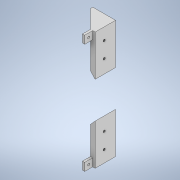
# Autodesk Inventor part: usb_battery_pocket_2
Saved by Autodesk Inventor 2021.3 (Build 253353010, 353A)
## iProperties
Created: 2021-10-31
Part Number: usb_battery_pocket_2
Material: Generic
Document SubType Name: Modeling
Designer: jesse
Density: 1 g/cm^3
Appearance: Default
Author: jesse
Autodesk Inventor part; units mm, degrees
ref_plane "YZ Plane" through (0, 0, 0) normal (1, 0, 0) x (0, 1, 0)
ref_plane "XZ Plane" through (0, 0, 0) normal (0, 1, 0) x (-1, 0, 0)
ref_plane "XY Plane" through (0, 0, 0) normal (0, 0, 1) x (1, 0, 0)
sketch "Sketch1" plane through (0, 0, 0) normal (0, 1, 0) x (-1, 0, 0)
  line L0 (0.4379, 4.9107) -> (0.4379, -5.0893)
  line L1 (0.4379, -5.0893) -> (-2.7621, -5.0893)
  line L2 (-2.7621, -5.0893) -> (-2.7621, -31.0893)
  line L3 (-2.7621, -31.0893) -> (26.2379, -31.0893)
  line L4 (26.2379, -31.0893) -> (26.2379, -28.0893)
  line L5 (26.2379, -28.0893) -> (0.2379, -28.0893)
  line L6 (0.2379, -28.0893) -> (0.2379, -8.0893)
  line L7 (0.2379, -8.0893) -> (3.2379, -8.0893)
  line L8 (3.2379, -8.0893) -> (3.2379, 4.9107)
  line L9 (3.2379, 4.9107) -> (0.4379, 4.9107)
  circle A0 centre (11.7379, -16.5893) radius 11.5
  line L10 (3.2379, -8.0893) -> (3.2379, -8.8433)
  line L11 (3.2379, -5.0893) -> (26.2379, -28.0893)
  point P0 (0, 0)
  point P1 (11.7379, -28.0893)
  point P2 (5.2457, -7.0971)
  dimension "d61" = 23
  dimension "d0" = 20
  dimension "d1" = 3
  dimension "d2" = 3
  dimension "d3" = 2.8
  dimension "d4" = 10
  dimension "d5" = 3
  dimension "d7" = 3.2
  dimension "d8" = 23
  constraints: 24 end point, 9 perpendicular, 3 vertical, 1 horizontal, 1 point on line, 3 other
  measures "d0" distance of L5.end L6.end
  measures "d1" distance between parallel lines of L2 L6
  measures "d2" distance between parallel lines of L7 L1
  measures "d3" distance between parallel lines of L0 L8
  measures "d4" distance of L0.start L0.end
  measures "d5" distance between parallel lines of L3 L5
  measures "d7" distance of L0.end L1.end
  measures "d8" horizontal distance of L11.start L4.end
extrude "Extrusion1" add sketch "Sketch1" along normal blind 150 contours L9 L8 L7 L6 L5 L4 L3 L2 L1 L0 | L11 A0 L10 L8 | L10 A0 L6 L7 | A0 L5 L6
sketch "Sketch2" plane through (2.7621, 0, -31.0893) normal (0, 0, -1) x (-1, 0, 0)
  line L0 (29, 0) -> (29, 150) projected
  line L1 (29, 130) -> (0, 98)
  line L2 (0, 0) -> (0, 150) projected
  line L3 (29, 20) -> (0, 52)
  line L4 (0, 0) -> (29, 0) projected
  point P0 (2.7621, 0)
  dimension "d11" = 20
  dimension "d12" = 20
  dimension "d13" = 32
  dimension "d14" = 32
  constraints: 4 end point, 4 point on line
  measures "d11" distance from line of L4 L3.start
  measures "d12" distance of L1.start L0.end
  measures "d13" vertical distance of L1.start L1.end
  measures "d14" vertical distance of L3.start L3.end
extrude "Extrusion2" cut sketch "Sketch2" against normal blind 150 contours L3 L2 L1 L0
sketch "Sketch3" plane through (-3.2379, 150, -5.0893) normal (-1, 0, 0) x (0, 0, 1)
  line L0 (0, 0) -> (10, 0) projected
  line L1 (0, -150) -> (0, -104.6207) projected
  line L2 (10, 0) -> (0, 0)
  line L3 (0, 0) -> (0, -150)
  line L4 (0, -150) -> (10, -150)
  line L5 (10, -150) -> (10, 0)
  line L6 (10, -48.469) -> (10, 0) projected
  line L7 (10, -10) -> (0, -10)
  line L8 (10, -150) -> (10, -104.6207) projected
  line L9 (10, -140) -> (0, -140)
  circle A0 centre (5, -5) radius 1.4
  circle A1 centre (5, -145) radius 1.4
  point P0 (5.0893, -150)
  point P1 (0, -140)
  dimension "d17" = 10
  dimension "d18" = 10
  dimension "d19" = 2.8
  dimension "d20" = 2.8
  dimension "d21" = 5
  dimension "d22" = 5
  dimension "d23" = 5
  dimension "d24" = 5
  constraints: 12 end point, 4 point on line, 3 perpendicular, 2 centre point, 2 parallel, 1 horizontal
  measures "d17" distance between parallel lines of L7 L0
  measures "d18" distance between parallel lines of L4 L9
  measures "d19" diameter of A0
  measures "d20" diameter of A1
  measures "d21" distance from line of L3 A0.centre
  measures "d22" distance from line of L0 A0.centre
  measures "d23" distance from line of L4 A1.centre
  measures "d24" distance from line of L1 A1.centre
extrude "Extrusion3" cut sketch "Sketch3" against normal blind 150 contours L7 L5 L9 L1 L3 | A0 | A1
sketch "Sketch5" plane through (2.7621, 150, -5.0893) normal (1, 0, 0) x (0, 0, -1)
  line L0 (2.0078, 0) -> (0, 0) projected
  line L1 (23, -36) -> (23, 0) projected
  line L2 (2.0078, 0) -> (23, 0)
  line L3 (23, 0) -> (23, -3)
  line L4 (23, -3) -> (2.0078, -3)
  line L5 (2.0078, -3) -> (2.0078, 0)
  line L6 (2.0078, -150) -> (2.0078, -106.8362) projected
  line L7 (23, -150) -> (23, -130) projected
  line L8 (2.0078, -150) -> (23, -150)
  line L9 (23, -150) -> (23, -147)
  line L10 (23, -147) -> (2.0078, -147)
  line L11 (2.0078, -147) -> (2.0078, -150)
  point P0 (-5.0893, -150)
  point P1 (2.0078, -147)
  dimension "d31" = 3
  dimension "d32" = 3
  constraints: 16 end point, 4 parallel, 2 horizontal, 2 perpendicular, 2 point on line
  measures "d31" distance between parallel lines of L2 L4
  measures "d32" distance between parallel lines of L10 L8
extrude "Extrusion5" add sketch "Sketch5" against normal up to surface (29 mm away)
sketch "Sketch6" plane through (0, 150, 0) normal (0, 1, 0) x (1, 0, 0)
  line L0 (-5.2457, 7.0971) -> (-26.2379, 7.0971) projected
  line L1 (-11.7379, 28.0893) -> (-26.2379, 28.0893) projected
  line L2 (-5.2457, 7.0971) -> (-26.2379, 28.0893)
  line L3 (-26.2379, 7.0971) -> (-26.2379, 28.0893)
  line L4 (-26.2379, 7.0971) -> (-5.2457, 7.0971)
  point P0 (0, 0)
  constraints: 6 end point, 1 collinear, 1 perpendicular
extrude "Extrusion6" cut sketch "Sketch6" against normal through all
sketch "Sketch7" plane through (2.7621, 150, -5.0893) normal (1, 0, 0) x (0, 0, -1)
  circle A0 centre (11.5, -15) radius 2.3
  circle A1 centre (11.5, -35) radius 2.3
  circle A2 centre (11.5, -115) radius 2.3
  circle A3 centre (11.5, -135) radius 2.3
  line L0 (0, -52) -> (0, 0) projected
  line L1 (0, -150) -> (0, -98) projected
  line L2 (0, -150) -> (26, -150) projected
  line L3 (0, 0) -> (26, 0) projected
  point P0 (-5.0893, -150)
  dimension "d37" = 4.6
  dimension "d38" = 4.6
  dimension "d39" = 4.6
  dimension "d40" = 4.6
  dimension "d41" = 11.5
  dimension "d42" = 11.5
  dimension "d43" = 11.5
  dimension "d44" = 11.5
  dimension "d45" = 15
  dimension "d46" = 20
  dimension "d47" = 20
  dimension "d48" = 15
  constraints: 4 centre point
  measures "d37" diameter of A2
  measures "d38" diameter of A3
  measures "d39" diameter of A0
  measures "d40" diameter of A1
  measures "d41" distance from line of L0 A1.centre
  measures "d42" distance from line of L0 A0.centre
  measures "d43" distance from line of L1 A2.centre
  measures "d44" distance from line of L1 A3.centre
  measures "d45" distance from line of A3.centre L2
  measures "d46" distance of A3.centre A2.centre
  measures "d47" distance of A1.centre A0.centre
  measures "d48" distance from line of L3 A0.centre
extrude "Extrusion7" cut sketch "Sketch7" against normal blind 150
sketch "Sketch8" plane through (2.7621, 150, -5.0893) normal (1, 0, 0) x (0, 0, -1)
  line L0 (0, 0) -> (26, 0) projected
  line L1 (0, -150) -> (0, -140) projected
  line L2 (26, 0) -> (0, 0)
  line L3 (0, 0) -> (0, -150)
  line L4 (0, -150) -> (26, -150)
  line L5 (26, -150) -> (26, 0)
  line L6 (26, -75) -> (0, -75)
  circle A0 centre (11.5, -135) radius 1.4
  circle A1 centre (11.5, -115) radius 1.4
  circle A2 centre (11.5, -115) radius 2.3 projected
  circle A3 centre (11.5, -135) radius 2.3 projected
  circle A4 centre (11.5, -35) radius 2.3 projected
  circle A5 centre (11.5, -35) radius 1.4
  circle A6 centre (11.5, -15) radius 1.4
  circle A7 centre (11.5, -15) radius 2.3 projected
  point P0 (-5.0893, -150)
  dimension "d55" = 2.8
  dimension "d56" = 2.8
  dimension "d57" = 2.8
  dimension "d58" = 2.8
  constraints: 10 end point, 4 centre point, 3 concentric, 2 midpoint, 2 parallel, 1 coincident, 1 horizontal, 1 perpendicular
  measures "d55" diameter of A0
  measures "d56" diameter of A1
  measures "d57" diameter of A5
  measures "d58" diameter of A6
extrude "Extrusion9" add sketch "Sketch8" against normal blind 0.6 contours A2 | A3 | A4 | A7
sketch "Sketch9" plane through (2.7621, 150, -31.0893) normal (0, 0, -1) x (-1, 0, 0)
  point P0 (2.7621, -150)
body "Solid1"
